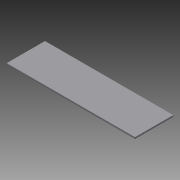
# Autodesk Inventor part: UNLHEP-14-01-P-010_WeightBlade
Saved by Autodesk Inventor 2013 (Build 170138000, 138)
## iProperties
Created: 2014-01-06
Part Number: UNLHEP-14-01-P-010_WeightBlade
Material: Allgemein
Document SubType Name: Modeling
Designer: Frank Meier
Density: 1 g/cm^3
Project: UNL Pixel Phase I
Author: Frank Meier
Autodesk Inventor part; units mm, degrees
ref_plane "YZ Plane" through (0, 0, 0) normal (1, 0, 0) x (0, 1, 0)
ref_plane "XZ Plane" through (0, 0, 0) normal (0, 1, 0) x (-1, 0, 0)
ref_plane "XY Plane" through (0, 0, 0) normal (0, 0, 1) x (1, 0, 0)
sketch "Skizze1" plane through (0, 0, 0) normal (0, 0, 1) x (1, 0, 0)
  line L0 (-33.5, -10) -> (33.5, -10)
  line L1 (33.5, -10) -> (33.5, 10)
  line L2 (33.5, 10) -> (-33.5, 10)
  line L3 (-33.5, 10) -> (-33.5, -10)
  line L4 (-33.5, -10) -> (33.5, 10) construction
  line L5 (33.5, -10) -> (-33.5, 10) construction
  point P0 (0, 0)
  dimension "d0" = 20
  dimension "d2" = 67
  constraints: 12 end point, 2 midpoint, 2 parallel, 1 horizontal, 1 perpendicular
  measures "d0" distance between parallel lines of L0 L2
  measures "d2" distance between parallel lines of L1 L3
extrude "Extrusion1" add sketch "Skizze1" along normal blind 0.8
